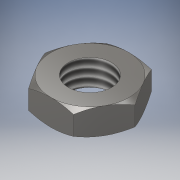
# Autodesk Inventor part: Door Plate Nut
Saved by Autodesk Inventor 2018 (Build 220112000, 112)
## iProperties
Created: 2016-10-27
Part Number: Door Plate Nut
Material: Steel, Carbon
Document SubType Name: Modeling
Designer: Joey
Density: 7.85 g/cm^3
Appearance: Semi-Polished
Mass: 166.052 g
Surface Area: 67.5398 cm^2
Volume: 21.1531 cm^3
Author: Joey
Autodesk Inventor part; units mm, degrees
ref_plane "YZ Plane" through (0, 0, 0) normal (1, 0, 0) x (0, 1, 0)
ref_plane "XZ Plane" through (0, 0, 0) normal (0, 1, 0) x (-1, 0, 0)
ref_plane "XY Plane" through (0, 0, 0) normal (0, 0, 1) x (1, 0, 0)
sketch "Sketch3" plane through (0, 0, 0) normal (0, 1, 0) x (-1, 0, 0)
  line L0 (10.9985, 0) -> (5.4993, -9.525)
  line L1 (5.4993, -9.525) -> (-5.4993, -9.525)
  line L2 (-5.4993, -9.525) -> (-10.9985, 0)
  line L3 (-10.9985, 0) -> (-5.4993, 9.525)
  line L4 (-5.4993, 9.525) -> (5.4993, 9.525)
  line L5 (5.4993, 9.525) -> (10.9985, 0)
  point P0 (0, 0)
  point P1 (0, 0)
  point P2 (0, 0)
  dimension "d27" = 19.05
  constraints: 12 end point, 2 coincident, 1 horizontal, 13 other
  measures "d27" distance between parallel lines of L4 L1
extrude "Extrusion2" add sketch "Sketch3" along normal mid plane 6.35
sketch "Sketch5" plane through (0, 0, 0) normal (0, 0, 1) x (1, 0, 0)
  line L0 (0, -8.89) -> (0, 8.89) projected
  line L1 (10.9985, 3.175) -> (5.4993, 3.175) construction
  line L2 (5.4993, 3.175) -> (5.4993, -3.175) projected
  line L3 (10.9985, 3.175) -> (5.4993, 3.175) projected
  line L4 (10.9985, 3.175) -> (10.9985, -3.175) construction
  line L5 (5.4993, -3.175) -> (10.9985, -3.175) projected
  line L6 (9.525, 3.175) -> (10.9985, 3.175)
  line L7 (10.9985, 3.175) -> (10.9985, 2.3243)
  line L8 (10.9985, 2.3243) -> (9.525, 3.175)
  line L9 (0, 0) -> (14.3088, 0) construction
  line L10 (9.525, -3.175) -> (10.9985, -3.175)
  line L11 (10.9985, -3.175) -> (10.9985, -2.3243)
  line L12 (10.9985, -2.3243) -> (9.525, -3.175)
  dimension "d15" = 19.05
  dimension "d16" = 30
  constraints: 14 end point, 3 symmetric about line, 2 collinear, 2 horizontal, 1 perpendicular
  measures "d15" diameter of L6.start L0
  measures "d16" angle of L8 L6
revolve "Revolution3" cut sketch "Sketch5" angle 360 about axis through (0, -10, 0) along (0, 1, 0)
hole "Hole1" at (0, 3.175, 0) direction (0, -1, 0) diameter 10.5918 end through all thread size "1/2-13 UNC" class "2B" standard "ANSI Unified Screw Threads"
equation "\"diameter\" = 25.4"
equation "\"length\" = 76.2"
body "Solid1"
